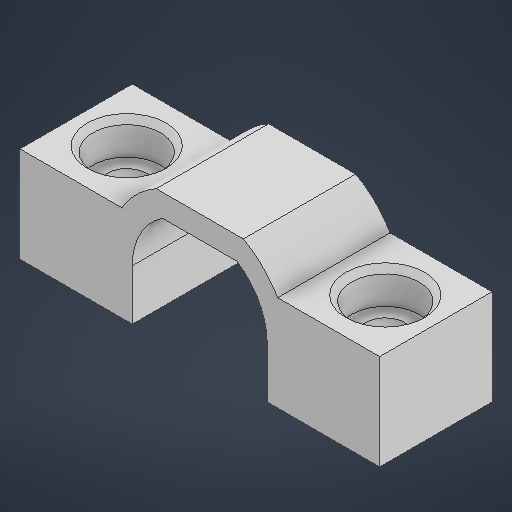
# Autodesk Inventor part: Držak motoru
Saved by Autodesk Inventor 2026 (Build 300175000, 175)
## iProperties
Created: 2025-04-28
Part Number: Držak motoru
Material: Všeobecné
Document SubType Name: Modeling
Designer: vadim
Density: 1 g/cm^3
Appearance: Výchozí
Author: vadim
Autodesk Inventor part; units mm, degrees
ref_plane "YZ Plane" through (0, 0, 0) normal (1, 0, 0) x (0, 1, 0)
ref_plane "XZ Plane" through (0, 0, 0) normal (0, 1, 0) x (-1, 0, 0)
sketch "Náčrt1" plane through (0, 0, 0) normal (0, 0, 1) x (1, 0, 0)
  line L0 (-3.3166, 5) -> (3.3166, 5)
  line L1 (3.3166, -5) -> (-3.3166, -5)
  arc A0 (-3.3166, 5) -> (-6, 0) centre (0, 0) ccw
  arc A1 (6, 0) -> (3.3166, 5) centre (0, 0) ccw
  line L2 (-3.3166, 5) -> (3.3166, -5)
  line L3 (3.3166, 5) -> (-3.3166, -5)
  line L4 (-16, 7) -> (16, 7)
  line L5 (16, 7) -> (16, -5)
  line L6 (16, -5) -> (-16, -5)
  line L7 (-16, -5) -> (-16, 7)
  line L8 (0, 5) -> (0, -5)
  line L9 (-16, 4) -> (-6.9282, 4)
  arc A2 (8, 0) -> (3.873, 7) centre (0, 0) ccw
  line L10 (3.873, 7) -> (-3.873, 7)
  line L11 (-8, 0) -> (-8, -5)
  line L12 (-6, 0) -> (-6, -5)
  line L13 (6, 0) -> (6, -5)
  line L14 (8, 0) -> (8, -5)
  arc A3 (-3.873, 7) -> (-8, 0) centre (0, 0) ccw
  line L15 (6.9282, 4) -> (16, 4)
  point P0 (3.873, 7)
  dimension "d13" = 10
  dimension "d14" = 12
  dimension "d15" = 6
  dimension "d16" = 32
  dimension "d17" = 12
  dimension "d20" = 9
  constraints: 32 end point, 10 point on circle, 7 point on line, 6 perpendicular, 4 centre point, 4 tangent, 3 horizontal, 3 parallel, 2 midpoint, 1 coincident, 1 collinear, 1 other
  measures "d13" distance between parallel lines of L1 L0
  measures "d14" distance of L12.start L13.start
  measures "d15" radius of A0
  measures "d16" distance of L5.end L6.end
  measures "d17" distance of L4.end L5.end
  measures "d20" distance between parallel lines of L6 L9
extrude "Vysunutí1" add sketch "Náčrt1" along normal blind 10 contours A0 L12 L6 L11 A3 L4 A2 L14 L13 A1 L0 | L6 L7 L9 A3 L11 | L14 A2 L15 L5 L6
sketch "Náčrt2" plane through (-16, 4, 0) normal (0, 1, 0) x (1, 0, 0)
  line L0 (0, 0) -> (0, -10) projected
  line L1 (9.0718, -10) -> (0, -10) projected
  point P0 (16, 0)
  point P1 (4.5, -5)
  dimension "d24" = 4.5
  dimension "d25" = 5
  measures "d24" distance from line of L0 point (4.5, -5)
  measures "d25" distance from line of L1 point (4.5, -5)
hole "Díra1" at (-11.5, 4, 5) direction (0, -1, 0) diameter 3.5 end through all counterbore diameter 6 counterbore depth 3
ref_plane "Pracovní rovina1" through (0, -5, 0) normal (1, 0, 0) x (0, 0, -1)
mirror "Zrcadlit1" about plane through (0, -5, 0) normal (1, 0, 0) of "Díra1"
move faces "Posunout1" translate (0, 0.5, 0) faces at (-7.2543, -5, 5.0703) (7.2543, -5, 5.0703)
chamfer "Zkosení1" distance 0.5 angle 45 2 edges at (-11.5, 4, 2) (11.5, 4, 2)
